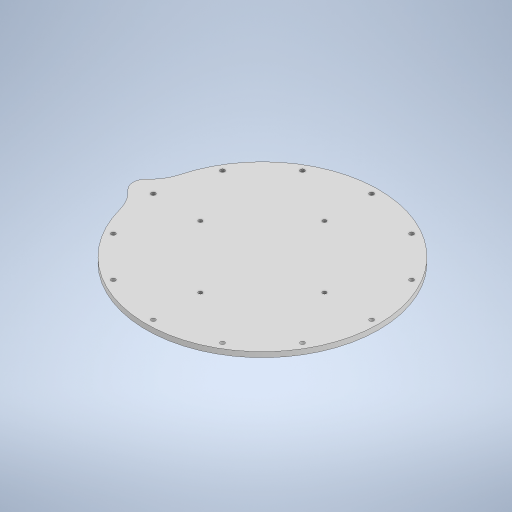
# Autodesk Inventor part: MDF Board
Saved by Autodesk Inventor 2024 (Build 280153000, 153)
## iProperties
Created: 2023-10-03
Part Number: MDF Board
Material: Generic
Document SubType Name: Modeling
Designer: komor
Density: 1 g/cm^3
Appearance: Default
Author: komor
Autodesk Inventor part; units mm, degrees
ref_plane "YZ Plane" through (0, 0, 0) normal (1, 0, 0) x (0, 1, 0)
ref_plane "XZ Plane" through (0, 0, 0) normal (0, 1, 0) x (-1, 0, 0)
ref_plane "XY Plane" through (0, 0, 0) normal (0, 0, 1) x (1, 0, 0)
sketch "Sketch1" plane through (0, 0, 0) normal (0, 1, 0) x (-1, 0, 0)
  arc A0 (-195.1682, -43.6963) -> (-195.1682, -43.6963) centre (0, 0) ccw construction
  spline S0 degree 3 poles (212.7614, 63.8524) (213.1534, 65.8524) (213.5259, 67.8561) (213.8787, 69.8633) knots 0 0 0 0 0.019635 0.019635 0.019635 0.019635 construction
  circle A1 centre (0, 0) radius 225
  line L0 (0, 0) -> (0, 120) construction
  line L1 (0, 0) -> (0, -120) construction
  line L2 (0, 0) -> (-120, 0) construction
  line L3 (0, 0) -> (120, 0) construction
  circle A2 centre (-120, 0) radius 3.5
  circle A3 centre (0, -120) radius 3.5
  circle A4 centre (120, 0) radius 3.5
  circle A5 centre (0, 120) radius 3.5
  circle A6 centre (0, -211.1656) radius 4
  circle A7 centre (105.5828, -182.8748) radius 4
  circle A8 centre (182.8748, -105.5828) radius 4
  circle A9 centre (211.1656, 0) radius 4
  circle A10 centre (182.8748, 105.5828) radius 4
  circle A11 centre (105.5828, 182.8748) radius 4
  circle A12 centre (0, 211.1656) radius 4
  circle A13 centre (-105.5828, 182.8748) radius 4
  circle A14 centre (-182.8748, 105.5828) radius 4
  circle A15 centre (-211.1656, 0) radius 4
  circle A16 centre (-182.8748, -105.5828) radius 4
  circle A17 centre (-105.5828, -182.8748) radius 4
  circle A18 centre (225, 0) radius 25
  line L4 (225, 0) -> (242.9975, 17.352)
  line L5 (225, 0) -> (250, 0)
  arc A19 (217.6933, 56.8737) -> (242.9975, 17.352) centre (295.1945, 78.633) ccw
  arc A20 (242.9975, -17.352) -> (217.6933, -56.8737) centre (295.1945, -78.633) ccw
  point P0 (217.6933, -56.8737)
  point P1 (242.9975, -17.352)
  dimension "d0" = 120
  dimension "d1" = 120
  dimension "d2" = 120
  dimension "d3" = 120
  dimension "d4" = 7
  dimension "d5" = 7
  dimension "d6" = 7
  dimension "d7" = 7
  dimension "d10" = 450
  dimension "d11" = 8
  dimension "d14" = 360
  dimension "d16" = 50
  dimension "d17" = 43.954
  constraints: 21 centre point, 12 end point, 11 point on circle, 5 coincident, 3 symmetric about line, 2 horizontal, 2 vertical, 1 perpendicular, 29 other
  measures "d0" distance of L0.start L0.end
  measures "d1" distance of L0.start L1.end
  measures "d2" distance of L0.start L2.end
  measures "d3" distance of L0.start L3.end
  measures "d4" diameter of A2
  measures "d5" diameter of A3
  measures "d6" diameter of A4
  measures "d7" diameter of A5
  measures "d10" diameter of A1
  measures "d11" diameter of A6
  measures "d16" diameter of A18
  measures "d17" angle of L5 L4
extrude "Extrusion1" add sketch "Sketch1" along normal blind 10 contours A1 A18 | A19 A18 A1 | A1 A18 A20 | A18 A19 L4 A1 | A1 A18 | A1 L5 A18 A20 | L4 A18 L5
body "Solid1"
